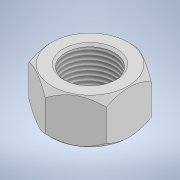
# Autodesk Inventor part: nut
Saved by Autodesk Inventor 2020 (Build 240168000, 168)
## iProperties
Created: 2022-11-14
Part Number: nut
Material: Generic
Document SubType Name: Modeling
Designer: Matthew Ng
Density: 1 g/cm^3
Appearance: Default
Author: Matthew Ng
Autodesk Inventor part; units mm, degrees
ref_plane "YZ Plane" through (0, 0, 0) normal (1, 0, 0) x (0, 1, 0)
ref_plane "XZ Plane" through (0, 0, 0) normal (0, 1, 0) x (-1, 0, 0)
sketch "Sketch1" plane through (0, 0, 0) normal (0, 1, 0) x (-1, 0, 0)
  line L0 (0, -10) -> (-8.6603, -5)
  line L1 (-8.6603, -5) -> (-8.6603, 5)
  line L2 (-8.6603, 5) -> (0, 10)
  line L3 (0, 10) -> (8.6603, 5)
  line L4 (8.6603, 5) -> (8.6603, -5)
  line L5 (8.6603, -5) -> (0, -10)
  point P0 (0, 0)
  point P1 (0, 0)
  dimension "d1" = 20
  constraints: 12 end point, 13 other
  measures "d1" distance of L2.end L0.start
extrude "Extrusion1" add sketch "Sketch1" along normal blind 10
sketch "Sketch2" plane through (0, 0, 0) normal (1, 0, 0) x (0, 1, 0)
  line L0 (10, -5) -> (10, -10) projected
  line L1 (10, -10) -> (8.5, -10)
  line L2 (10, -8.5) -> (10, -10)
  line L3 (8.5, -10) -> (10, -8.5)
  line L4 (-2, 0) -> (12, 0) projected
  point P0 (0, 0)
  constraints: 6 end point, 1 horizontal
revolve "Revolution1" cut sketch "Sketch2" angle 360 about axis through (0, -10, 0) along (0, 1, 0)
ref_plane "Work Plane1" through (0, 5, 0) normal (0, 1, 0) x (1, 0, 0)
mirror "Mirror1" about plane through (0, 5, 0) normal (0, 1, 0) of "Revolution1"
sketch "Sketch3" plane through (0, 10, 0) normal (0, 1, 0) x (1, 0, 0)
  circle A0 centre (0, 0) radius 8.5 projected
  constraints: 1 coincident
hole "Hole1" at (0, 10, 0) direction (0, -1, 0) diameter 10.917 depth 29.1 tip angle 118 thread size "M12x1" class "6H" standard "ISO Metric profile"
chamfer "Chamfer1" distance 0.5 angle 45 2 edges at (0, 10, -5.4585) (0, 0, -5.4585)
body "Solid1"
